Autodesk Inventor part; units mm, degrees
(part 6 of 8)
  arc A393 (19.9886, 4.7302) -> (19.9233, 4.7694) centre (19.956, 4.7498) ccw
  arc A394 (19.3814, 3.8663) -> (19.4467, 3.8271) centre (19.414, 3.8467) ccw
  line L135 (19.9559, 4.7498) -> (19.9559, 3.1242)
  arc A395 (19.9178, 3.1242) -> (19.994, 3.1242) centre (19.9559, 3.1242) ccw
  arc A396 (19.994, 4.7498) -> (19.9178, 4.7498) centre (19.9559, 4.7498) ccw
  line L136 (20.7656, 3.5758) -> (20.7656, 4.2982)
  arc A397 (20.8037, 4.2982) -> (20.7275, 4.2982) centre (20.7656, 4.2982) ccw
  arc A398 (20.7275, 3.5758) -> (20.8037, 3.5758) centre (20.7656, 3.5758) ccw
  arc A399 (21.6687, 4.2982) -> (20.7656, 4.2982) centre (21.2172, 4.2982) ccw
  arc A400 (21.6306, 4.2982) -> (21.7068, 4.2982) centre (21.6687, 4.2982) ccw
  arc A401 (20.7275, 4.2982) -> (20.8037, 4.2982) centre (20.7656, 4.2982) ccw
  line L137 (21.6687, 4.2982) -> (21.6687, 3.5758)
  arc A402 (21.6306, 3.5758) -> (21.7068, 3.5758) centre (21.6687, 3.5758) ccw
  arc A403 (21.7068, 4.2982) -> (21.6306, 4.2982) centre (21.6687, 4.2982) ccw
  arc A404 (20.7656, 3.5758) -> (21.6687, 3.5758) centre (21.2172, 3.5758) ccw
  arc A405 (20.8037, 3.5758) -> (20.7275, 3.5758) centre (20.7656, 3.5758) ccw
  arc A406 (21.7068, 3.5758) -> (21.6306, 3.5758) centre (21.6687, 3.5758) ccw
  line L138 (21.4881, 3.4854) -> (21.8493, 3.1242)
  arc A407 (21.8224, 3.0973) -> (21.8762, 3.1511) centre (21.8493, 3.1242) ccw
  arc A408 (21.515, 3.5124) -> (21.4611, 3.4585) centre (21.4881, 3.4855) ccw
  line L139 (22.6584, 4.7498) -> (22.2972, 3.4854)
  arc A409 (22.2605, 3.4959) -> (22.3338, 3.475) centre (22.2972, 3.4855) ccw
  arc A410 (22.6951, 4.7393) -> (22.6218, 4.7603) centre (22.6585, 4.7498) ccw
  line L140 (22.2972, 3.4854) -> (23.2003, 3.4854)
  arc A411 (23.2003, 3.4473) -> (23.2003, 3.5235) centre (23.2003, 3.4854) ccw
  arc A412 (22.2972, 3.5235) -> (22.2972, 3.4473) centre (22.2972, 3.4854) ccw
  line L141 (22.9293, 3.8467) -> (22.9293, 3.1242)
  arc A413 (22.8912, 3.1242) -> (22.9674, 3.1242) centre (22.9293, 3.1242) ccw
  arc A414 (22.9674, 3.8467) -> (22.8912, 3.8467) centre (22.9293, 3.8467) ccw
  line L142 (40.4622, 2.9972) -> (40.4622, 4.6228)
  arc A415 (40.5003, 4.6228) -> (40.4241, 4.6228) centre (40.4622, 4.6228) ccw
  arc A416 (40.4241, 2.9972) -> (40.5003, 2.9972) centre (40.4622, 2.9972) ccw
  line L143 (40.4622, 3.9003) -> (41.3653, 3.9003)
  arc A417 (41.3653, 3.8622) -> (41.3653, 3.9384) centre (41.3653, 3.9003) ccw
  arc A418 (40.4622, 3.9384) -> (40.4622, 3.8622) centre (40.4622, 3.9003) ccw
  line L144 (41.3653, 4.6228) -> (41.3653, 2.9972)
  arc A419 (41.3272, 2.9972) -> (41.4034, 2.9972) centre (41.3653, 2.9972) ccw
  arc A420 (41.4034, 4.6228) -> (41.3272, 4.6228) centre (41.3653, 4.6228) ccw
  line L145 (42.1295, 4.6228) -> (42.1295, 3.4488)
  arc A421 (42.0914, 3.4488) -> (42.1676, 3.4488) centre (42.1295, 3.4488) ccw
  arc A422 (42.1676, 4.6228) -> (42.0914, 4.6228) centre (42.1295, 4.6228) ccw
  arc A423 (42.1295, 3.4488) -> (43.0326, 3.4488) centre (42.5811, 3.4488) ccw
  arc A424 (42.1676, 3.4488) -> (42.0914, 3.4488) centre (42.1295, 3.4488) ccw
  arc A425 (43.0707, 3.4488) -> (42.9945, 3.4488) centre (43.0326, 3.4488) ccw
  line L146 (43.0326, 3.4488) -> (43.0326, 4.6228)
  arc A426 (43.0707, 4.6228) -> (42.9945, 4.6228) centre (43.0326, 4.6228) ccw
  arc A427 (42.9945, 3.4488) -> (43.0707, 3.4488) centre (43.0326, 3.4488) ccw
  line L147 (43.8108, 2.9972) -> (43.8108, 4.6228)
  arc A428 (43.8489, 4.6228) -> (43.7727, 4.6228) centre (43.8108, 4.6228) ccw
  arc A429 (43.7727, 2.9972) -> (43.8489, 2.9972) centre (43.8108, 2.9972) ccw
  line L148 (43.8108, 4.6228) -> (44.3526, 3.7197)
  arc A430 (44.32, 3.7001) -> (44.3853, 3.7393) centre (44.3527, 3.7197) ccw
  arc A431 (43.8434, 4.6424) -> (43.7781, 4.6032) centre (43.8107, 4.6228) ccw
  line L149 (44.3526, 3.7197) -> (44.8945, 4.6228)
  arc A432 (44.9272, 4.6032) -> (44.8618, 4.6424) centre (44.8945, 4.6228) ccw
  arc A433 (44.32, 3.7393) -> (44.3853, 3.7001) centre (44.3527, 3.7197) ccw
  line L150 (44.8945, 4.6228) -> (44.8945, 2.9972)
  arc A434 (44.8564, 2.9972) -> (44.9326, 2.9972) centre (44.8945, 2.9972) ccw
  arc A435 (44.9326, 4.6228) -> (44.8564, 4.6228) centre (44.8945, 4.6228) ccw
  line L151 (62.3062, 4.2418) -> (62.8481, 2.6162)
  arc A436 (62.8119, 2.6042) -> (62.8842, 2.6282) centre (62.8481, 2.6162) ccw
  arc A437 (62.3423, 4.2538) -> (62.2701, 4.2298) centre (62.3062, 4.2418) ccw
  line L152 (62.8481, 2.6162) -> (63.3899, 4.2418)
  arc A438 (63.4261, 4.2298) -> (63.3538, 4.2538) centre (63.3899, 4.2418) ccw
  arc A439 (62.8119, 2.6282) -> (62.8842, 2.6042) centre (62.8481, 2.6162) ccw
  line L153 (64.0986, 4.2418) -> (64.0986, 2.6162)
  arc A440 (64.0605, 2.6162) -> (64.1367, 2.6162) centre (64.0986, 2.6162) ccw
  arc A441 (64.1367, 4.2418) -> (64.0605, 4.2418) centre (64.0986, 4.2418) ccw
  line L154 (63.9179, 2.6162) -> (64.2792, 2.6162)
  arc A442 (64.2792, 2.5781) -> (64.2792, 2.6543) centre (64.2792, 2.6162) ccw
  arc A443 (63.9179, 2.6543) -> (63.9179, 2.5781) centre (63.9179, 2.6162) ccw
  line L155 (63.9179, 4.2418) -> (64.2792, 4.2418)
  arc A444 (64.2792, 4.2037) -> (64.2792, 4.2799) centre (64.2792, 4.2418) ccw
  arc A445 (63.9179, 4.2799) -> (63.9179, 4.2037) centre (63.9179, 4.2418) ccw
  line L156 (64.9707, 3.5193) -> (65.4223, 3.5193)
  arc A446 (65.4223, 3.4812) -> (65.4223, 3.5574) centre (65.4223, 3.5193) ccw
  arc A447 (64.9707, 3.5574) -> (64.9707, 3.4812) centre (64.9707, 3.5193) ccw
  arc A448 (65.4223, 2.6162) -> (65.4223, 3.5193) centre (65.4223, 3.0678) ccw
  arc A449 (65.4223, 2.6543) -> (65.4223, 2.5781) centre (65.4223, 2.6162) ccw
  arc A450 (65.4223, 3.5574) -> (65.4223, 3.4812) centre (65.4223, 3.5193) ccw
  line L157 (65.4223, 2.6162) -> (64.9707, 2.6162)
  arc A451 (64.9707, 2.6543) -> (64.9707, 2.5781) centre (64.9707, 2.6162) ccw
  arc A452 (65.4223, 2.5781) -> (65.4223, 2.6543) centre (65.4223, 2.6162) ccw
  line L158 (64.9707, 2.6162) -> (64.9707, 4.2418)
  arc A453 (65.0088, 4.2418) -> (64.9326, 4.2418) centre (64.9707, 4.2418) ccw
  arc A454 (64.9326, 2.6162) -> (65.0088, 2.6162) centre (64.9707, 2.6162) ccw
  line L159 (64.9707, 4.2418) -> (65.4223, 4.2418)
  arc A455 (65.4223, 4.2037) -> (65.4223, 4.2799) centre (65.4223, 4.2418) ccw
  arc A456 (64.9707, 4.2799) -> (64.9707, 4.2037) centre (64.9707, 4.2418) ccw
  arc A457 (65.4223, 3.5193) -> (65.4223, 4.2418) centre (65.4223, 3.8805) ccw
  arc A458 (65.4223, 3.5574) -> (65.4223, 3.4812) centre (65.4223, 3.5193) ccw
  arc A459 (65.4223, 4.2799) -> (65.4223, 4.2037) centre (65.4223, 4.2418) ccw
  arc A460 (84.4381, 2.6162) -> (84.7993, 2.9774) centre (84.4381, 2.9774) ccw
  arc A461 (84.4381, 2.6543) -> (84.4381, 2.5781) centre (84.4381, 2.6162) ccw
  arc A462 (84.8374, 2.9774) -> (84.7612, 2.9774) centre (84.7993, 2.9774) ccw
  arc A463 (83.8962, 2.842) -> (84.4381, 2.6162) centre (84.4381, 3.3794) ccw
  arc A464 (83.9233, 2.8688) -> (83.8691, 2.8151) centre (83.8962, 2.8419) ccw
  arc A465 (84.4381, 2.5781) -> (84.4381, 2.6543) centre (84.4381, 2.6162) ccw
  arc A466 (84.3026, 4.2418) -> (83.9414, 3.8806) centre (84.3026, 3.8806) ccw
  arc A467 (84.3026, 4.2037) -> (84.3026, 4.2799) centre (84.3026, 4.2418) ccw
  arc A468 (83.9033, 3.8806) -> (83.9795, 3.8806) centre (83.9414, 3.8806) ccw
  arc A469 (84.709, 4.1063) -> (84.3026, 4.2418) centre (84.3026, 3.5645) ccw
  arc A470 (84.6861, 4.0759) -> (84.7319, 4.1368) centre (84.709, 4.1063) ccw
  arc A471 (84.3026, 4.2799) -> (84.3026, 4.2037) centre (84.3026, 4.2418) ccw
  arc A472 (83.9414, 3.8806) -> (84.122, 3.5645) centre (84.3082, 3.8806) ccw
  arc A473 (83.9795, 3.8806) -> (83.9033, 3.8806) centre (83.9414, 3.8806) ccw
  arc A474 (84.1026, 3.5316) -> (84.1413, 3.5973) centre (84.1219, 3.5644) ccw
  arc A475 (84.7993, 2.9774) -> (84.6187, 3.2935) centre (84.4325, 2.9774) ccw
  arc A476 (84.7612, 2.9774) -> (84.8374, 2.9774) centre (84.7993, 2.9774) ccw
  arc A477 (84.638, 3.3264) -> (84.5993, 3.2607) centre (84.6187, 3.2936) ccw
  line L160 (84.6187, 3.2935) -> (84.122, 3.5645)
  arc A478 (84.1402, 3.5979) -> (84.1037, 3.531) centre (84.1219, 3.5644) ccw
  arc A479 (84.6004, 3.2601) -> (84.6369, 3.327) centre (84.6187, 3.2936) ccw
  line L161 (85.4623, 4.2418) -> (85.4623, 2.6162)
  arc A480 (85.4242, 2.6162) -> (85.5004, 2.6162) centre (85.4623, 2.6162) ccw
  arc A481 (85.5004, 4.2418) -> (85.4242, 4.2418) centre (85.4623, 4.2418) ccw
  line L162 (85.4623, 2.6162) -> (86.1848, 2.6162)
  arc A482 (86.1848, 2.5781) -> (86.1848, 2.6543) centre (86.1848, 2.6162) ccw
  arc A483 (85.4623, 2.6543) -> (85.4623, 2.5781) centre (85.4623, 2.6162) ccw
  line L163 (86.6716, 4.2418) -> (87.2135, 3.4742)
  arc A484 (87.1824, 3.4522) -> (87.2446, 3.4961) centre (87.2135, 3.4742) ccw
  arc A485 (86.7027, 4.2638) -> (86.6405, 4.2198) centre (86.6716, 4.2418) ccw
  line L164 (87.2135, 3.4742) -> (87.7553, 4.2418)
  arc A486 (87.7865, 4.2198) -> (87.7242, 4.2638) centre (87.7553, 4.2418) ccw
  arc A487 (87.1824, 3.4961) -> (87.2446, 3.4522) centre (87.2135, 3.4742) ccw
  line L165 (87.2135, 2.6162) -> (87.2135, 3.4742)
  arc A488 (87.2516, 3.4742) -> (87.1754, 3.4742) centre (87.2135, 3.4742) ccw
  arc A489 (87.1754, 2.6162) -> (87.2516, 2.6162) centre (87.2135, 2.6162) ccw
  line L166 (59.2187, 22.9362) -> (58.8574, 22.9362)
  arc A490 (58.8574, 22.9743) -> (58.8574, 22.8981) centre (58.8574, 22.9362) ccw
  arc A491 (59.2187, 22.8981) -> (59.2187, 22.9743) centre (59.2187, 22.9362) ccw
  arc A492 (58.4962, 23.2974) -> (58.8574, 22.9362) centre (58.8574, 23.2974) ccw
  arc A493 (58.5343, 23.2974) -> (58.4581, 23.2974) centre (58.4962, 23.2974) ccw
  arc A494 (58.8574, 22.8981) -> (58.8574, 22.9743) centre (58.8574, 22.9362) ccw
  line L167 (58.4962, 23.2974) -> (58.4962, 24.2006)
  arc A495 (58.5343, 24.2006) -> (58.4581, 24.2006) centre (58.4962, 24.2006) ccw
  arc A496 (58.4581, 23.2974) -> (58.5343, 23.2974) centre (58.4962, 23.2974) ccw
  arc A497 (58.8574, 24.5618) -> (58.4962, 24.2006) centre (58.8574, 24.2006) ccw
  arc A498 (58.8574, 24.5237) -> (58.8574, 24.5999) centre (58.8574, 24.5618) ccw
  arc A499 (58.4581, 24.2006) -> (58.5343, 24.2006) centre (58.4962, 24.2006) ccw
  line L168 (58.8574, 24.5618) -> (59.2187, 24.5618)
  arc A500 (59.2187, 24.5237) -> (59.2187, 24.5999) centre (59.2187, 24.5618) ccw
  arc A501 (58.8574, 24.5999) -> (58.8574, 24.5237) centre (58.8574, 24.5618) ccw
  line L169 (59.8028, 23.3878) -> (59.8028, 24.1102)
  arc A502 (59.8409, 24.1102) -> (59.7647, 24.1102) centre (59.8028, 24.1102) ccw
  arc A503 (59.7647, 23.3878) -> (59.8409, 23.3878) centre (59.8028, 23.3878) ccw
  arc A504 (60.7059, 24.1102) -> (59.8028, 24.1102) centre (60.2544, 24.1102) ccw
  arc A505 (60.6678, 24.1102) -> (60.744, 24.1102) centre (60.7059, 24.1102) ccw
  arc A506 (59.7647, 24.1102) -> (59.8409, 24.1102) centre (59.8028, 24.1102) ccw
  line L170 (60.7059, 24.1102) -> (60.7059, 23.3878)
  arc A507 (60.6678, 23.3878) -> (60.744, 23.3878) centre (60.7059, 23.3878) ccw
  arc A508 (60.744, 24.1102) -> (60.6678, 24.1102) centre (60.7059, 24.1102) ccw
  arc A509 (59.8027, 23.3878) -> (60.7059, 23.3878) centre (60.2543, 23.3878) ccw
  arc A510 (59.8408, 23.3878) -> (59.7646, 23.3878) centre (59.8027, 23.3878) ccw
  arc A511 (60.744, 23.3878) -> (60.6678, 23.3878) centre (60.7059, 23.3878) ccw
  line L171 (61.418, 22.9362) -> (61.418, 24.5618)
  arc A512 (61.4561, 24.5618) -> (61.3799, 24.5618) centre (61.418, 24.5618) ccw
  arc A513 (61.3799, 22.9362) -> (61.4561, 22.9362) centre (61.418, 22.9362) ccw
  line L172 (61.418, 24.5618) -> (62.3211, 22.9362)
  arc A514 (62.2878, 22.9177) -> (62.3544, 22.9547) centre (62.3211, 22.9362) ccw
  arc A515 (61.4513, 24.5803) -> (61.3847, 24.5433) centre (61.418, 24.5618) ccw
  line L173 (62.3211, 22.9362) -> (62.3211, 24.5618)
  arc A516 (62.3592, 24.5618) -> (62.283, 24.5618) centre (62.3211, 24.5618) ccw
  arc A517 (62.283, 22.9362) -> (62.3592, 22.9362) centre (62.3211, 22.9362) ccw
  line L174 (63.0853, 22.9362) -> (63.0853, 24.5618)
  arc A518 (63.1234, 24.5618) -> (63.0472, 24.5618) centre (63.0853, 24.5618) ccw
  arc A519 (63.0472, 22.9362) -> (63.1234, 22.9362) centre (63.0853, 22.9362) ccw
  line L175 (63.0853, 24.5618) -> (63.9884, 22.9362)
  arc A520 (63.9551, 22.9177) -> (64.0217, 22.9547) centre (63.9884, 22.9362) ccw
  arc A521 (63.1186, 24.5803) -> (63.052, 24.5433) centre (63.0853, 24.5618) ccw
  line L176 (63.9884, 22.9362) -> (63.9884, 24.5618)
  arc A522 (64.0265, 24.5618) -> (63.9503, 24.5618) centre (63.9884, 24.5618) ccw
  arc A523 (63.9503, 22.9362) -> (64.0265, 22.9362) centre (63.9884, 22.9362) ccw
  line L177 (65.4781, 22.9362) -> (64.7556, 22.9362)
  arc A524 (64.7556, 22.9743) -> (64.7556, 22.8981) centre (64.7556, 22.9362) ccw
  arc A525 (65.4781, 22.8981) -> (65.4781, 22.9743) centre (65.4781, 22.9362) ccw
  line L178 (64.7556, 22.9362) -> (64.7556, 24.5618)
  arc A526 (64.7937, 24.5618) -> (64.7175, 24.5618) centre (64.7556, 24.5618) ccw
  arc A527 (64.7175, 22.9362) -> (64.7937, 22.9362) centre (64.7556, 22.9362) ccw
  line L179 (64.7556, 24.5618) -> (65.4781, 24.5618)
  arc A528 (65.4781, 24.5237) -> (65.4781, 24.5999) centre (65.4781, 24.5618) ccw
  arc A529 (64.7556, 24.5999) -> (64.7556, 24.5237) centre (64.7556, 24.5618) ccw
  line L180 (64.7556, 23.8393) -> (65.2975, 23.8393)
  arc A530 (65.2975, 23.8012) -> (65.2975, 23.8774) centre (65.2975, 23.8393) ccw
  arc A531 (64.7556, 23.8774) -> (64.7556, 23.8012) centre (64.7556, 23.8393) ccw
  line L181 (66.7738, 22.9362) -> (66.4125, 22.9362)
  arc A532 (66.4125, 22.9743) -> (66.4125, 22.8981) centre (66.4125, 22.9362) ccw
  arc A533 (66.7738, 22.8981) -> (66.7738, 22.9743) centre (66.7738, 22.9362) ccw
  arc A534 (66.0513, 23.2974) -> (66.4125, 22.9362) centre (66.4125, 23.2974) ccw
  arc A535 (66.0894, 23.2974) -> (66.0132, 23.2974) centre (66.0513, 23.2974) ccw
  arc A536 (66.4125, 22.8981) -> (66.4125, 22.9743) centre (66.4125, 22.9362) ccw
  line L182 (66.0513, 23.2974) -> (66.0513, 24.2006)
  arc A537 (66.0894, 24.2006) -> (66.0132, 24.2006) centre (66.0513, 24.2006) ccw
  arc A538 (66.0132, 23.2974) -> (66.0894, 23.2974) centre (66.0513, 23.2974) ccw
  arc A539 (66.4125, 24.5618) -> (66.0513, 24.2006) centre (66.4125, 24.2006) ccw
  arc A540 (66.4125, 24.5237) -> (66.4125, 24.5999) centre (66.4125, 24.5618) ccw
  arc A541 (66.0132, 24.2006) -> (66.0894, 24.2006) centre (66.0513, 24.2006) ccw
  line L183 (66.4125, 24.5618) -> (66.7738, 24.5618)
  arc A542 (66.7738, 24.5237) -> (66.7738, 24.5999) centre (66.7738, 24.5618) ccw
  arc A543 (66.4125, 24.5999) -> (66.4125, 24.5237) centre (66.4125, 24.5618) ccw
  line L184 (67.7052, 22.9362) -> (67.7052, 24.5618)
  arc A544 (67.7433, 24.5618) -> (67.6671, 24.5618) centre (67.7052, 24.5618) ccw
  arc A545 (67.6671, 22.9362) -> (67.7433, 22.9362) centre (67.7052, 22.9362) ccw
  line L185 (67.2536, 24.5618) -> (68.1568, 24.5618)
  arc A546 (68.1568, 24.5237) -> (68.1568, 24.5999) centre (68.1568, 24.5618) ccw
  arc A547 (67.2536, 24.5999) -> (67.2536, 24.5237) centre (67.2536, 24.5618) ccw
  line L186 (68.7126, 23.3878) -> (68.7126, 24.1102)
  arc A548 (68.7507, 24.1102) -> (68.6745, 24.1102) centre (68.7126, 24.1102) ccw
  arc A549 (68.6745, 23.3878) -> (68.7507, 23.3878) centre (68.7126, 23.3878) ccw
  arc A550 (69.6157, 24.1102) -> (68.7126, 24.1102) centre (69.1642, 24.1102) ccw
  arc A551 (69.5776, 24.1102) -> (69.6538, 24.1102) centre (69.6157, 24.1102) ccw
  arc A552 (68.6745, 24.1102) -> (68.7507, 24.1102) centre (68.7126, 24.1102) ccw
  line L187 (69.6157, 24.1102) -> (69.6157, 23.3878)
  arc A553 (69.5776, 23.3878) -> (69.6538, 23.3878) centre (69.6157, 23.3878) ccw
  arc A554 (69.6538, 24.1102) -> (69.5776, 24.1102) centre (69.6157, 24.1102) ccw
  arc A555 (68.7126, 23.3878) -> (69.6157, 23.3878) centre (69.1642, 23.3878) ccw
  arc A556 (68.7507, 23.3878) -> (68.6745, 23.3878) centre (68.7126, 23.3878) ccw
  arc A557 (69.6538, 23.3878) -> (69.5776, 23.3878) centre (69.6157, 23.3878) ccw
  line L188 (70.3369, 22.9362) -> (70.3369, 24.5618)
  arc A558 (70.375, 24.5618) -> (70.2988, 24.5618) centre (70.3369, 24.5618) ccw
  arc A559 (70.2988, 22.9362) -> (70.375, 22.9362) centre (70.3369, 22.9362) ccw
  line L189 (70.3369, 24.5618) -> (70.7885, 24.5618)
  arc A560 (70.7885, 24.5237) -> (70.7885, 24.5999) centre (70.7885, 24.5618) ccw
  arc A561 (70.3369, 24.5999) -> (70.3369, 24.5237) centre (70.3369, 24.5618) ccw
  arc A562 (70.7885, 23.6587) -> (70.7885, 24.5618) centre (70.7885, 24.1103) ccw
  arc A563 (70.7885, 23.6968) -> (70.7885, 23.6206) centre (70.7885, 23.6587) ccw
  arc A564 (70.7885, 24.5999) -> (70.7885, 24.5237) centre (70.7885, 24.5618) ccw
  line L190 (70.7885, 23.6587) -> (70.3369, 23.6587)
  arc A565 (70.3369, 23.6968) -> (70.3369, 23.6206) centre (70.3369, 23.6587) ccw
  arc A566 (70.7885, 23.6206) -> (70.7885, 23.6968) centre (70.7885, 23.6587) ccw
  line L191 (71.24, 22.9362) -> (70.8788, 23.6587)
  arc A567 (70.9129, 23.6757) -> (70.8447, 23.6416) centre (70.8788, 23.6587) ccw
  arc A568 (71.206, 22.9192) -> (71.2741, 22.9532) centre (71.24, 22.9362) ccw
  arc A569 (72.3807, 22.9362) -> (72.7419, 23.2974) centre (72.3807, 23.2974) ccw
  arc A570 (72.3807, 22.9743) -> (72.3807, 22.8981) centre (72.3807, 22.9362) ccw
  arc A571 (72.78, 23.2974) -> (72.7038, 23.2974) centre (72.7419, 23.2974) ccw
  arc A572 (71.8388, 23.162) -> (72.3807, 22.9362) centre (72.3807, 23.6994) ccw
  arc A573 (71.8659, 23.1888) -> (71.8118, 23.1351) centre (71.8388, 23.1619) ccw
  arc A574 (72.3807, 22.8981) -> (72.3807, 22.9743) centre (72.3807, 22.9362) ccw
  arc A575 (72.2452, 24.5618) -> (71.884, 24.2006) centre (72.2452, 24.2006) ccw
  arc A576 (72.2452, 24.5237) -> (72.2452, 24.5999) centre (72.2452, 24.5618) ccw
  arc A577 (71.8459, 24.2006) -> (71.9221, 24.2006) centre (71.884, 24.2006) ccw
  arc A578 (72.6516, 24.4263) -> (72.2452, 24.5618) centre (72.2452, 23.8845) ccw
  arc A579 (72.6287, 24.3959) -> (72.6745, 24.4568) centre (72.6516, 24.4263) ccw
  arc A580 (72.2452, 24.5999) -> (72.2452, 24.5237) centre (72.2452, 24.5618) ccw
  arc A581 (71.884, 24.2006) -> (72.0646, 23.8845) centre (72.2508, 24.2006) ccw
  arc A582 (71.9221, 24.2006) -> (71.8459, 24.2006) centre (71.884, 24.2006) ccw
  arc A583 (72.0452, 23.8516) -> (72.0839, 23.9173) centre (72.0645, 23.8845) ccw
  arc A584 (72.7419, 23.2974) -> (72.5613, 23.6135) centre (72.3751, 23.2974) ccw
  arc A585 (72.7038, 23.2974) -> (72.78, 23.2974) centre (72.7419, 23.2974) ccw
  arc A586 (72.5806, 23.6464) -> (72.5419, 23.5807) centre (72.5613, 23.6136) ccw
  line L192 (72.5613, 23.6135) -> (72.0646, 23.8845)
  arc A587 (72.0828, 23.9179) -> (72.0463, 23.851) centre (72.0645, 23.8845) ccw
  arc A588 (72.543, 23.5801) -> (72.5795, 23.647) centre (72.5613, 23.6136) ccw
  line L193 (73.3498, 24.2006) -> (73.8014, 24.5618)
  arc A589 (73.8252, 24.532) -> (73.7776, 24.5916) centre (73.8014, 24.5618) ccw
  arc A590 (73.326, 24.2303) -> (73.3736, 24.1708) centre (73.3498, 24.2005) ccw
  line L194 (73.8014, 24.5618) -> (73.8014, 22.9362)
  arc A591 (73.7633, 22.9362) -> (73.8395, 22.9362) centre (73.8014, 22.9362) ccw
  arc A592 (73.8395, 24.5618) -> (73.7633, 24.5618) centre (73.8014, 24.5618) ccw
  line L195 (73.3498, 22.9362) -> (74.2529, 22.9362)
  arc A593 (74.2529, 22.8981) -> (74.2529, 22.9743) centre (74.2529, 22.9362) ccw
  arc A594 (73.3498, 22.9743) -> (73.3498, 22.8981) centre (73.3498, 22.9362) ccw
  line L196 (74.8469, 22.7556) -> (75.5694, 22.7556)
  arc A595 (75.5694, 22.7175) -> (75.5694, 22.7937) centre (75.5694, 22.7556) ccw
  arc A596 (74.8469, 22.7937) -> (74.8469, 22.7175) centre (74.8469, 22.7556) ccw
  arc A597 (76.6532, 22.9362) -> (77.0144, 23.2974) centre (76.6532, 23.2974) ccw
  arc A598 (76.6532, 22.9743) -> (76.6532, 22.8981) centre (76.6532, 22.9362) ccw
  arc A599 (77.0525, 23.2974) -> (76.9763, 23.2974) centre (77.0144, 23.2974) ccw
  arc A600 (76.1113, 23.162) -> (76.6532, 22.9362) centre (76.6532, 23.6994) ccw
  arc A601 (76.1384, 23.1888) -> (76.0843, 23.1351) centre (76.1113, 23.1619) ccw
  arc A602 (76.6532, 22.8981) -> (76.6532, 22.9743) centre (76.6532, 22.9362) ccw
  arc A603 (76.5177, 24.5618) -> (76.1565, 24.2006) centre (76.5177, 24.2006) ccw
  arc A604 (76.5177, 24.5237) -> (76.5177, 24.5999) centre (76.5177, 24.5618) ccw
  arc A605 (76.1184, 24.2006) -> (76.1946, 24.2006) centre (76.1565, 24.2006) ccw
  arc A606 (76.9241, 24.4263) -> (76.5177, 24.5618) centre (76.5177, 23.8845) ccw
  arc A607 (76.9013, 24.3959) -> (76.947, 24.4568) centre (76.9241, 24.4263) ccw
  arc A608 (76.5177, 24.5999) -> (76.5177, 24.5237) centre (76.5177, 24.5618) ccw
  arc A609 (76.1565, 24.2006) -> (76.3371, 23.8845) centre (76.5233, 24.2006) ccw
  arc A610 (76.1946, 24.2006) -> (76.1184, 24.2006) centre (76.1565, 24.2006) ccw
  arc A611 (76.3178, 23.8516) -> (76.3565, 23.9173) centre (76.3372, 23.8845) ccw
  arc A612 (77.0144, 23.2974) -> (76.8338, 23.6135) centre (76.6476, 23.2974) ccw
  arc A613 (76.9763, 23.2974) -> (77.0525, 23.2974) centre (77.0144, 23.2974) ccw
  arc A614 (76.8532, 23.6464) -> (76.8145, 23.5807) centre (76.8338, 23.6136) ccw
  line L197 (76.8338, 23.6135) -> (76.3371, 23.8845)
  arc A615 (76.3554, 23.9179) -> (76.3189, 23.851) centre (76.3372, 23.8845) ccw
  arc A616 (76.8156, 23.5801) -> (76.8521, 23.647) centre (76.8338, 23.6136) ccw
  line L198 (78.3999, 22.9362) -> (77.6774, 22.9362)
  arc A617 (77.6774, 22.9743) -> (77.6774, 22.8981) centre (77.6774, 22.9362) ccw
  arc A618 (78.3999, 22.8981) -> (78.3999, 22.9743) centre (78.3999, 22.9362) ccw
  line L199 (77.6774, 22.9362) -> (77.6774, 24.5618)
  arc A619 (77.7155, 24.5618) -> (77.6393, 24.5618) centre (77.6774, 24.5618) ccw
  arc A620 (77.6393, 22.9362) -> (77.7155, 22.9362) centre (77.6774, 22.9362) ccw
  line L200 (77.6774, 24.5618) -> (78.3999, 24.5618)
  arc A621 (78.3999, 24.5237) -> (78.3999, 24.5999) centre (78.3999, 24.5618) ccw
  arc A622 (77.6774, 24.5999) -> (77.6774, 24.5237) centre (77.6774, 24.5618) ccw
  line L201 (77.6774, 23.8393) -> (78.2193, 23.8393)
  arc A623 (78.2193, 23.8012) -> (78.2193, 23.8774) centre (78.2193, 23.8393) ccw
  arc A624 (77.6774, 23.8774) -> (77.6774, 23.8012) centre (77.6774, 23.8393) ccw
  line L202 (79.0292, 22.9362) -> (79.0292, 24.5618)
  arc A625 (79.0673, 24.5618) -> (78.9911, 24.5618) centre (79.0292, 24.5618) ccw
  arc A626 (78.9911, 22.9362) -> (79.0673, 22.9362) centre (79.0292, 22.9362) ccw
  line L203 (79.0292, 24.5618) -> (79.9323, 22.9362)
  arc A627 (79.899, 22.9177) -> (79.9656, 22.9547) centre (79.9323, 22.9362) ccw
  arc A628 (79.0625, 24.5803) -> (78.9959, 24.5433) centre (79.0292, 24.5618) ccw
  line L204 (79.9323, 22.9362) -> (79.9323, 24.5618)
  arc A629 (79.9704, 24.5618) -> (79.8942, 24.5618) centre (79.9323, 24.5618) ccw
  arc A630 (79.8942, 22.9362) -> (79.9704, 22.9362) centre (79.9323, 22.9362) ccw
  arc A631 (81.1342, 22.9362) -> (81.4954, 23.2974) centre (81.1342, 23.2974) ccw
  arc A632 (81.1342, 22.9743) -> (81.1342, 22.8981) centre (81.1342, 22.9362) ccw
  arc A633 (81.5335, 23.2974) -> (81.4573, 23.2974) centre (81.4954, 23.2974) ccw
  arc A634 (80.5923, 23.162) -> (81.1342, 22.9362) centre (81.1342, 23.6994) ccw
  arc A635 (80.6193, 23.1888) -> (80.5652, 23.1351) centre (80.5923, 23.162) ccw
  arc A636 (81.1342, 22.8981) -> (81.1342, 22.9743) centre (81.1342, 22.9362) ccw
  arc A637 (80.9987, 24.5618) -> (80.6374, 24.2006) centre (80.9987, 24.2005) ccw
  arc A638 (80.9987, 24.5237) -> (80.9987, 24.5999) centre (80.9987, 24.5618) ccw
  arc A639 (80.5993, 24.2006) -> (80.6755, 24.2006) centre (80.6374, 24.2006) ccw
  arc A640 (81.4051, 24.4263) -> (80.9987, 24.5618) centre (80.9987, 23.8845) ccw
  arc A641 (81.3822, 24.3959) -> (81.428, 24.4568) centre (81.4051, 24.4263) ccw
  arc A642 (80.9987, 24.5999) -> (80.9987, 24.5237) centre (80.9987, 24.5618) ccw
  arc A643 (80.6374, 24.2006) -> (80.8181, 23.8845) centre (81.0043, 24.2006) ccw
  arc A644 (80.6755, 24.2006) -> (80.5993, 24.2006) centre (80.6374, 24.2006) ccw
  arc A645 (80.7987, 23.8516) -> (80.8374, 23.9173) centre (80.8181, 23.8845) ccw
  arc A646 (81.4954, 23.2974) -> (81.3148, 23.6135) centre (81.1286, 23.2974) ccw
  arc A647 (81.4573, 23.2974) -> (81.5335, 23.2974) centre (81.4954, 23.2974) ccw
  arc A648 (81.3341, 23.6464) -> (81.2954, 23.5807) centre (81.3148, 23.6136) ccw
  line L205 (81.3148, 23.6135) -> (80.8181, 23.8845)
  arc A649 (80.8363, 23.9179) -> (80.7998, 23.851) centre (80.8181, 23.8845) ccw
  arc A650 (81.2965, 23.5801) -> (81.333, 23.647) centre (81.3148, 23.6136) ccw
  line L206 (82.1033, 23.3878) -> (82.1033, 24.1102)
  arc A651 (82.1414, 24.1102) -> (82.0652, 24.1102) centre (82.1033, 24.1102) ccw
  arc A652 (82.0652, 23.3878) -> (82.1414, 23.3878) centre (82.1033, 23.3878) ccw
  arc A653 (83.0064, 24.1102) -> (82.1033, 24.1102) centre (82.5549, 24.1102) ccw
  arc A654 (82.9683, 24.1102) -> (83.0445, 24.1102) centre (83.0064, 24.1102) ccw
  arc A655 (82.0652, 24.1102) -> (82.1414, 24.1102) centre (82.1033, 24.1102) ccw
  line L207 (83.0064, 24.1102) -> (83.0064, 23.3878)
  arc A656 (82.9683, 23.3878) -> (83.0445, 23.3878) centre (83.0064, 23.3878) ccw
  arc A657 (83.0445, 24.1102) -> (82.9683, 24.1102) centre (83.0064, 24.1102) ccw
  arc A658 (82.1033, 23.3878) -> (83.0064, 23.3878) centre (82.5549, 23.3878) ccw
  arc A659 (82.1414, 23.3878) -> (82.0652, 23.3878) centre (82.1033, 23.3878) ccw
  arc A660 (83.0445, 23.3878) -> (82.9683, 23.3878) centre (83.0064, 23.3878) ccw
  arc A661 (29.4833, 24.1102) -> (29.5595, 24.1102) centre (29.5214, 24.1102) ccw
  arc A662 (30.3864, 24.1102) -> (30.4626, 24.1102) centre (30.4245, 24.1102) ccw
  arc A663 (30.4245, 24.1102) -> (29.5214, 24.1102) centre (29.9729, 24.1102) ccw
  arc A664 (29.4833, 23.3878) -> (29.5595, 23.3878) centre (29.5214, 23.3878) ccw
  arc A665 (29.5595, 24.1102) -> (29.4833, 24.1102) centre (29.5214, 24.1102) ccw
  line L208 (29.5214, 23.3878) -> (29.5214, 24.1102)
  arc A666 (28.483, 24.5999) -> (28.483, 24.5237) centre (28.483, 24.5618) ccw
  arc A667 (28.483, 23.8774) -> (28.483, 23.8012) centre (28.483, 23.8393) ccw
  arc A668 (28.483, 23.8393) -> (28.483, 24.5618) centre (28.483, 24.2005) ccw
  arc A669 (28.0315, 24.5999) -> (28.0315, 24.5237) centre (28.0315, 24.5618) ccw
  arc A670 (28.483, 24.5237) -> (28.483, 24.5999) centre (28.483, 24.5618) ccw
  line L209 (28.0315, 24.5618) -> (28.483, 24.5618)
  arc A671 (27.9934, 22.9362) -> (28.0696, 22.9362) centre (28.0315, 22.9362) ccw
  arc A672 (28.0696, 24.5618) -> (27.9934, 24.5618) centre (28.0315, 24.5618) ccw
  line L210 (28.0315, 22.9362) -> (28.0315, 24.5618)
  arc A673 (28.483, 22.8981) -> (28.483, 22.9743) centre (28.483, 22.9362) ccw
  arc A674 (28.0315, 22.9743) -> (28.0315, 22.8981) centre (28.0315, 22.9362) ccw
  line L211 (28.483, 22.9362) -> (28.0315, 22.9362)
  arc A675 (28.483, 23.8774) -> (28.483, 23.8012) centre (28.483, 23.8393) ccw
  arc A676 (28.483, 22.9743) -> (28.483, 22.8981) centre (28.483, 22.9362) ccw
  arc A677 (28.483, 22.9362) -> (28.483, 23.8393) centre (28.483, 23.3878) ccw
  arc A678 (28.0315, 23.8774) -> (28.0315, 23.8012) centre (28.0315, 23.8393) ccw
  arc A679 (28.483, 23.8012) -> (28.483, 23.8774) centre (28.483, 23.8393) ccw
  line L212 (28.0315, 23.8393) -> (28.483, 23.8393)
  arc A680 (27.3364, 23.3878) -> (27.2602, 23.3878) centre (27.2983, 23.3878) ccw
  arc A681 (26.4333, 23.3878) -> (26.3571, 23.3878) centre (26.3952, 23.3878) ccw
  arc A682 (26.3952, 23.3878) -> (27.2983, 23.3878) centre (26.8468, 23.3878) ccw
  arc A683 (27.3364, 24.1102) -> (27.2602, 24.1102) centre (27.2983, 24.1102) ccw
  arc A684 (27.2602, 23.3878) -> (27.3364, 23.3878) centre (27.2983, 23.3878) ccw
  line L213 (27.2983, 24.1102) -> (27.2983, 23.3878)
  arc A685 (26.3571, 24.1102) -> (26.4333, 24.1102) centre (26.3952, 24.1102) ccw
  arc A686 (27.2602, 24.1102) -> (27.3364, 24.1102) centre (27.2983, 24.1102) ccw
  arc A687 (27.2983, 24.1102) -> (26.3952, 24.1102) centre (26.8468, 24.1102) ccw
  arc A688 (26.3571, 23.3878) -> (26.4333, 23.3878) centre (26.3952, 23.3878) ccw
  arc A689 (26.4333, 24.1102) -> (26.3571, 24.1102) centre (26.3952, 24.1102) ccw
  line L214 (26.3952, 23.3878) -> (26.3952, 24.1102)
  arc A690 (25.7102, 22.9192) -> (25.7784, 22.9532) centre (25.7443, 22.9362) ccw
  arc A691 (25.4171, 23.6757) -> (25.349, 23.6416) centre (25.3831, 23.6587) ccw
  line L215 (25.7443, 22.9362) -> (25.3831, 23.6587)
  arc A692 (25.2928, 23.6206) -> (25.2928, 23.6968) centre (25.2928, 23.6587) ccw
  arc A693 (24.8412, 23.6968) -> (24.8412, 23.6206) centre (24.8412, 23.6587) ccw
  line L216 (25.2928, 23.6587) -> (24.8412, 23.6587)
  arc A694 (25.2928, 24.5999) -> (25.2928, 24.5237) centre (25.2928, 24.5618) ccw
  arc A695 (25.2928, 23.6968) -> (25.2928, 23.6206) centre (25.2928, 23.6587) ccw
  arc A696 (25.2928, 23.6587) -> (25.2928, 24.5618) centre (25.2928, 24.1103) ccw
  arc A697 (24.8412, 24.5999) -> (24.8412, 24.5237) centre (24.8412, 24.5618) ccw
  arc A698 (25.2928, 24.5237) -> (25.2928, 24.5999) centre (25.2928, 24.5618) ccw
  line L217 (24.8412, 24.5618) -> (25.2928, 24.5618)
  arc A699 (24.8031, 22.9362) -> (24.8793, 22.9362) centre (24.8412, 22.9362) ccw
  arc A700 (24.8793, 24.5618) -> (24.8031, 24.5618) centre (24.8412, 24.5618) ccw
  line L218 (24.8412, 22.9362) -> (24.8412, 24.5618)
  arc A701 (88.3801, 23.3045) -> (88.3801, 23.3807) centre (88.3801, 23.3426) ccw
  arc A702 (87.5673, 23.3807) -> (87.5673, 23.3045) centre (87.5673, 23.3426) ccw
  line L219 (88.3801, 23.3426) -> (87.5673, 23.3426)
  arc A703 (88.0098, 24.5738) -> (87.9375, 24.5498) centre (87.9736, 24.5618) ccw
  arc A704 (88.4794, 22.9242) -> (88.5517, 22.9482) centre (88.5155, 22.9362) ccw
  line L220 (87.9737, 24.5618) -> (88.5156, 22.9362)
  arc A705 (87.3957, 22.9482) -> (87.468, 22.9242) centre (87.4318, 22.9362) ccw
  arc A706 (88.0098, 24.5498) -> (87.9375, 24.5738) centre (87.9736, 24.5618) ccw
  line L221 (87.4318, 22.9362) -> (87.9737, 24.5618)
  arc A707 (86.5768, 24.5999) -> (86.5768, 24.5237) centre (86.5768, 24.5618) ccw
  arc A708 (86.9381, 24.5237) -> (86.9381, 24.5999) centre (86.9381, 24.5618) ccw
  line L222 (86.5768, 24.5618) -> (86.9381, 24.5618)
  arc A709 (86.1775, 24.2006) -> (86.2537, 24.2006) centre (86.2156, 24.2006) ccw
  arc A710 (86.5768, 24.5237) -> (86.5768, 24.5999) centre (86.5768, 24.5618) ccw
  arc A711 (86.5768, 24.5618) -> (86.2156, 24.2006) centre (86.5768, 24.2006) ccw
  arc A712 (86.1775, 23.2974) -> (86.2537, 23.2974) centre (86.2156, 23.2974) ccw
  arc A713 (86.2537, 24.2006) -> (86.1775, 24.2006) centre (86.2156, 24.2006) ccw
  line L223 (86.2156, 23.2974) -> (86.2156, 24.2006)
  arc A714 (86.5768, 22.8981) -> (86.5768, 22.9743) centre (86.5768, 22.9362) ccw
  arc A715 (86.2537, 23.2974) -> (86.1775, 23.2974) centre (86.2156, 23.2974) ccw
  arc A716 (86.2156, 23.2974) -> (86.5768, 22.9362) centre (86.5768, 23.2974) ccw
  arc A717 (86.9381, 22.8981) -> (86.9381, 22.9743) centre (86.9381, 22.9362) ccw
  arc A718 (86.5768, 22.9743) -> (86.5768, 22.8981) centre (86.5768, 22.9362) ccw
  line L224 (86.9381, 22.9362) -> (86.5768, 22.9362)
  arc A719 (85.24, 24.5999) -> (85.24, 24.5237) centre (85.24, 24.5618) ccw
  arc A720 (85.6012, 24.5237) -> (85.6012, 24.5999) centre (85.6012, 24.5618) ccw
  line L225 (85.24, 24.5618) -> (85.6012, 24.5618)
  arc A721 (85.24, 22.9743) -> (85.24, 22.8981) centre (85.24, 22.9362) ccw
  arc A722 (85.6012, 22.8981) -> (85.6012, 22.9743) centre (85.6012, 22.9362) ccw
  line L226 (85.24, 22.9362) -> (85.6012, 22.9362)
  arc A723 (85.4587, 24.5618) -> (85.3825, 24.5618) centre (85.4206, 24.5618) ccw
  arc A724 (85.3825, 22.9362) -> (85.4587, 22.9362) centre (85.4206, 22.9362) ccw
  line L227 (85.4206, 24.5618) -> (85.4206, 22.9362)
  arc A725 (84.5967, 22.9192) -> (84.6649, 22.9532) centre (84.6308, 22.9362) ccw
  arc A726 (84.3036, 23.6757) -> (84.2355, 23.6416) centre (84.2696, 23.6587) ccw
  line L228 (84.6308, 22.9362) -> (84.2696, 23.6587)
  arc A727 (84.1792, 23.6206) -> (84.1792, 23.6968) centre (84.1792, 23.6587) ccw
  arc A728 (83.7277, 23.6968) -> (83.7277, 23.6206) centre (83.7277, 23.6587) ccw
  line L229 (84.1792, 23.6587) -> (83.7277, 23.6587)
  arc A729 (84.1792, 24.5999) -> (84.1792, 24.5237) centre (84.1792, 24.5618) ccw
  arc A730 (84.1792, 23.6968) -> (84.1792, 23.6206) centre (84.1792, 23.6587) ccw
  arc A731 (84.1792, 23.6587) -> (84.1792, 24.5618) centre (84.1792, 24.1103) ccw
  arc A732 (83.7277, 24.5999) -> (83.7277, 24.5237) centre (83.7277, 24.5618) ccw
  arc A733 (84.1792, 24.5237) -> (84.1792, 24.5999) centre (84.1792, 24.5618) ccw
  line L230 (83.7277, 24.5618) -> (84.1792, 24.5618)
  arc A734 (83.6896, 22.9362) -> (83.7658, 22.9362) centre (83.7277, 22.9362) ccw
  arc A735 (83.7658, 24.5618) -> (83.6896, 24.5618) centre (83.7277, 24.5618) ccw
  line L231 (83.7277, 22.9362) -> (83.7277, 24.5618)
  arc A736 (14.1986, 26.9875) -> (14.4526, 27.2415) centre (14.1986, 27.2415) ccw
  arc A737 (14.1986, 27.0192) -> (14.1986, 26.9558) centre (14.1986, 26.9875) ccw
  arc A738 (14.4844, 27.2415) -> (14.4208, 27.2415) centre (14.4526, 27.2415) ccw
  arc A739 (13.8176, 27.1463) -> (14.1986, 26.9875) centre (14.1987, 27.5241) ccw
  arc A740 (13.8401, 27.1686) -> (13.7951, 27.1239) centre (13.8176, 27.1463) ccw
  arc A741 (14.1986, 26.9558) -> (14.1986, 27.0192) centre (14.1986, 26.9875) ccw
  arc A742 (14.1034, 28.1305) -> (13.8494, 27.8765) centre (14.1034, 27.8765) ccw
  arc A743 (14.1034, 28.0988) -> (14.1034, 28.1623) centre (14.1034, 28.1306) ccw
  arc A744 (13.8176, 27.8765) -> (13.8811, 27.8765) centre (13.8494, 27.8765) ccw
  arc A745 (14.3891, 28.0353) -> (14.1034, 28.1305) centre (14.1035, 27.6544) ccw
  arc A746 (14.37, 28.0099) -> (14.4082, 28.0606) centre (14.3891, 28.0353) ccw
  arc A747 (14.1033, 28.1623) -> (14.1034, 28.0988) centre (14.1034, 28.1306) ccw
  arc A748 (13.8494, 27.8765) -> (13.9764, 27.6543) centre (14.1073, 27.8765) ccw
  arc A749 (13.8811, 27.8765) -> (13.8176, 27.8765) centre (13.8494, 27.8765) ccw
  arc A750 (13.9602, 27.6269) -> (13.9925, 27.6816) centre (13.9764, 27.6543) ccw
  arc A751 (14.4526, 27.2415) -> (14.3256, 27.4638) centre (14.1946, 27.2415) ccw
  arc A752 (14.4208, 27.2415) -> (14.4844, 27.2415) centre (14.4526, 27.2415) ccw
  arc A753 (14.3417, 27.4911) -> (14.3095, 27.4364) centre (14.3256, 27.4638) ccw
  line L232 (14.3256, 27.4638) -> (13.9764, 27.6543)
  arc A754 (13.9916, 27.6821) -> (13.9611, 27.6264) centre (13.9764, 27.6543) ccw
  arc A755 (14.3104, 27.4359) -> (14.3408, 27.4916) centre (14.3256, 27.4638) ccw
  line L233 (14.859, 28.1305) -> (15.24, 26.9875)
  arc A756 (15.2099, 26.9775) -> (15.2701, 26.9975) centre (15.24, 26.9875) ccw
  arc A757 (14.8891, 28.1405) -> (14.8289, 28.1205) centre (14.859, 28.1305) ccw
  line L234 (15.24, 26.9875) -> (15.621, 28.1305)
  arc A758 (15.6511, 28.1205) -> (15.5909, 28.1405) centre (15.621, 28.1305) ccw
  arc A759 (15.2099, 26.9975) -> (15.2701, 26.9775) centre (15.24, 26.9875) ccw
  line L235 (16.0655, 27.8765) -> (16.383, 28.1305)
  arc A760 (16.4028, 28.1057) -> (16.3632, 28.1553) centre (16.383, 28.1305) ccw
  arc A761 (32.5995, 30.1046) -> (32.5487, 30.1046) centre (32.5741, 30.1046) ccw
  arc A762 (16.0457, 27.9013) -> (16.0853, 27.8517) centre (16.0655, 27.8765) ccw
  line L236 (16.383, 28.1305) -> (16.383, 26.9875)
  arc A763 (16.3513, 26.9875) -> (16.4147, 26.9875) centre (16.383, 26.9875) ccw
  arc A764 (16.4147, 28.1305) -> (16.3513, 28.1305) centre (16.383, 28.1305) ccw
  line L237 (16.0655, 26.9875) -> (16.7005, 26.9875)
  arc A765 (16.7005, 26.9558) -> (16.7005, 27.0192) centre (16.7005, 26.9875) ccw
  arc A766 (16.0655, 27.0192) -> (16.0655, 26.9558) centre (16.0655, 26.9875) ccw
  arc A767 (58.219, 30.4546) -> (58.219, 30.4038) centre (58.219, 30.4292) ccw
  arc A768 (32.5487, 29.5854) -> (32.5995, 29.5854) centre (32.5741, 29.5854) ccw
  arc A769 (49.8475, 27.1145) -> (50.1015, 27.3685) centre (49.8475, 27.3685) ccw
  arc A770 (49.8475, 27.1462) -> (49.8475, 27.0828) centre (49.8475, 27.1145) ccw
  arc A771 (50.1333, 27.3685) -> (50.0697, 27.3685) centre (50.1015, 27.3685) ccw
  arc A772 (49.4665, 27.2733) -> (49.8475, 27.1145) centre (49.8476, 27.6511) ccw
  arc A773 (49.489, 27.2956) -> (49.444, 27.2509) centre (49.4665, 27.2733) ccw
  arc A774 (49.8475, 27.0828) -> (49.8475, 27.1462) centre (49.8475, 27.1145) ccw
  arc A775 (49.7523, 28.2575) -> (49.4983, 28.0035) centre (49.7523, 28.0035) ccw
  arc A776 (49.7523, 28.2258) -> (49.7523, 28.2892) centre (49.7523, 28.2575) ccw
  arc A777 (49.4665, 28.0035) -> (49.53, 28.0035) centre (49.4983, 28.0035) ccw
  arc A778 (50.038, 28.1623) -> (49.7523, 28.2575) centre (49.7524, 27.7814) ccw
  arc A779 (50.0189, 28.1369) -> (50.0571, 28.1876) centre (50.038, 28.1623) ccw
  arc A780 (49.7522, 28.2892) -> (49.7523, 28.2258) centre (49.7523, 28.2575) ccw
  arc A781 (49.4983, 28.0035) -> (49.6253, 27.7813) centre (49.7562, 28.0035) ccw
  arc A782 (49.53, 28.0035) -> (49.4665, 28.0035) centre (49.4983, 28.0035) ccw
  arc A783 (49.6091, 27.7539) -> (49.6414, 27.8086) centre (49.6252, 27.7812) ccw
  arc A784 (50.1015, 27.3685) -> (49.9745, 27.5907) centre (49.8436, 27.3685) ccw
  arc A785 (50.0697, 27.3685) -> (50.1333, 27.3685) centre (50.1015, 27.3685) ccw
  arc A786 (49.9906, 27.6181) -> (49.9584, 27.5634) centre (49.9745, 27.5907) ccw
  line L238 (49.9745, 27.5907) -> (49.6253, 27.7813)
  arc A787 (49.6405, 27.8091) -> (49.61, 27.7534) centre (49.6252, 27.7812) ccw
  arc A788 (49.9593, 27.5629) -> (49.9897, 27.6186) centre (49.9745, 27.5907) ccw
  line L239 (50.5079, 28.2575) -> (50.8889, 27.1145)
  arc A789 (50.8588, 27.1045) -> (50.919, 27.1245) centre (50.8889, 27.1145) ccw
  arc A790 (50.538, 28.2675) -> (50.4778, 28.2475) centre (50.5079, 28.2575) ccw
  line L240 (50.8889, 27.1145) -> (51.2699, 28.2575)
  arc A791 (51.3, 28.2475) -> (51.2398, 28.2675) centre (51.2699, 28.2575) ccw
  arc A792 (50.8588, 27.1245) -> (50.919, 27.1045) centre (50.8889, 27.1145) ccw
  arc A793 (52.3494, 27.9718) -> (52.0637, 28.2575) centre (52.0637, 27.9718) ccw
  arc A794 (52.3177, 27.9718) -> (52.3812, 27.9718) centre (52.3494, 27.9718) ccw
  arc A795 (52.0637, 28.2892) -> (52.0637, 28.2258) centre (52.0637, 28.2575) ccw
  arc A796 (52.0637, 28.2575) -> (51.7144, 28.0035) centre (52.0637, 27.8904) ccw
  arc A797 (52.0636, 28.2258) -> (52.0637, 28.2892) centre (52.0637, 28.2575) ccw
  arc A798 (51.6842, 28.0133) -> (51.7446, 27.9937) centre (51.7144, 28.0035) ccw
  arc A799 (52.2542, 27.7495) -> (52.3494, 27.9718) centre (52.0425, 27.9717) ccw
  arc A800 (52.2323, 27.7725) -> (52.276, 27.7265) centre (52.2542, 27.7495) ccw
  arc A801 (52.3811, 27.9718) -> (52.3177, 27.9717) centre (52.3494, 27.9718) ccw
  line L241 (52.2542, 27.7495) -> (51.7144, 27.1145)
  arc A802 (51.6902, 27.1351) -> (51.7386, 27.0939) centre (51.7144, 27.1145) ccw
  arc A803 (52.2783, 27.7289) -> (52.23, 27.7701) centre (52.2542, 27.7495) ccw
  line L242 (51.7144, 27.1145) -> (52.3494, 27.1145)
  arc A804 (52.3494, 27.0828) -> (52.3494, 27.1462) centre (52.3494, 27.1145) ccw
  arc A805 (51.7144, 27.1462) -> (51.7144, 27.0828) centre (51.7144, 27.1145) ccw
  arc A806 (32.5995, 29.5854) -> (32.5487, 29.5854) centre (32.5741, 29.5854) ccw
  arc A807 (33.2486, 29.5854) -> (33.1978, 29.5854) centre (33.2232, 29.5854) ccw
  line L243 (33.7552, 30.4292) -> (33.7552, 29.5854)
  arc A808 (33.7298, 29.5854) -> (33.7806, 29.5854) centre (33.7552, 29.5854) ccw
  arc A809 (33.7806, 30.4292) -> (33.7298, 30.4292) centre (33.7552, 30.4292) ccw
  arc A810 (33.7552, 29.5854) -> (34.4043, 29.5854) centre (34.0798, 29.5854) ccw
  arc A811 (33.7806, 29.5854) -> (33.7298, 29.5854) centre (33.7552, 29.5854) ccw
  arc A812 (34.4297, 29.5854) -> (34.3789, 29.5854) centre (34.4043, 29.5854) ccw
  line L244 (34.4043, 29.5854) -> (34.4043, 30.4292)
  arc A813 (34.4297, 30.4292) -> (34.3789, 30.4292) centre (34.4043, 30.4292) ccw
  arc A814 (34.3789, 29.5854) -> (34.4297, 29.5854) centre (34.4043, 29.5854) ccw
  line L245 (35.1846, 29.2608) -> (35.1846, 30.4292)
  arc A815 (35.21, 30.4292) -> (35.1592, 30.4292) centre (35.1846, 30.4292) ccw
  arc A816 (35.1592, 29.2608) -> (35.21, 29.2608) centre (35.1846, 29.2608) ccw
  line L246 (34.8601, 30.4292) -> (35.5092, 30.4292)
  arc A817 (35.5092, 30.4038) -> (35.5092, 30.4546) centre (35.5092, 30.4292) ccw
  arc A818 (34.8601, 30.4546) -> (34.8601, 30.4038) centre (34.8601, 30.4292) ccw
  arc A819 (33.2232, 30.1046) -> (32.5741, 30.1046) centre (32.8987, 30.1046) ccw
  arc A820 (33.1978, 30.1046) -> (33.2486, 30.1046) centre (33.2232, 30.1046) ccw
  arc A821 (32.5487, 30.1046) -> (32.5995, 30.1046) centre (32.5741, 30.1046) ccw
  line L247 (33.2232, 30.1046) -> (33.2232, 29.5854)
  arc A822 (33.1978, 29.5854) -> (33.2486, 29.5854) centre (33.2232, 29.5854) ccw
  arc A823 (33.2486, 30.1046) -> (33.1978, 30.1046) centre (33.2232, 30.1046) ccw
  arc A824 (32.5741, 29.5854) -> (33.2232, 29.5854) centre (32.8987, 29.5854) ccw
  line L248 (32.5741, 29.5854) -> (32.5741, 30.1046)
  arc A825 (32.0167, 29.2608) -> (32.0675, 29.2608) centre (32.0421, 29.2608) ccw
  arc A826 (32.0675, 30.4292) -> (32.0167, 30.4292) centre (32.0421, 30.4292) ccw
  line L249 (32.0421, 29.2608) -> (32.0421, 30.4292)
  arc A827 (31.4152, 30.4415) -> (31.3708, 30.4169) centre (31.393, 30.4292) ccw
  arc A828 (32.0199, 29.2485) -> (32.0643, 29.2731) centre (32.0421, 29.2608) ccw
  line L250 (31.393, 30.4292) -> (32.0421, 29.2608)
  arc A829 (31.3676, 29.2608) -> (31.4184, 29.2608) centre (31.393, 29.2608) ccw
  arc A830 (31.4184, 30.4292) -> (31.3676, 30.4292) centre (31.393, 30.4292) ccw
  line L251 (31.393, 29.2608) -> (31.393, 30.4292)
  arc A831 (30.6352, 30.4546) -> (30.6352, 30.4038) centre (30.6352, 30.4292) ccw
  arc A832 (30.8949, 30.4038) -> (30.8949, 30.4546) centre (30.8949, 30.4292) ccw
  line L252 (30.6352, 30.4292) -> (30.8949, 30.4292)
  arc A833 (30.6352, 29.2862) -> (30.6352, 29.2354) centre (30.6352, 29.2608) ccw
  arc A834 (30.8949, 29.2354) -> (30.8949, 29.2862) centre (30.8949, 29.2608) ccw
  line L253 (30.6352, 29.2608) -> (30.8949, 29.2608)
  arc A835 (30.7905, 30.4292) -> (30.7397, 30.4292) centre (30.7651, 30.4292) ccw
  arc A836 (30.7397, 29.2608) -> (30.7905, 29.2608) centre (30.7651, 29.2608) ccw
  line L254 (30.7651, 30.4292) -> (30.7651, 29.2608)
  arc A837 (30.1117, 29.5854) -> (30.1625, 29.5854) centre (30.1371, 29.5854) ccw
  arc A838 (30.1625, 30.4292) -> (30.1117, 30.4292) centre (30.1371, 30.4292) ccw
  line L255 (30.1371, 29.5854) -> (30.1371, 30.4292)
  arc A839 (30.1625, 29.5854) -> (30.1117, 29.5854) centre (30.1371, 29.5854) ccw
  arc A840 (29.5134, 29.5854) -> (29.4626, 29.5854) centre (29.488, 29.5854) ccw
  arc A841 (29.488, 29.5854) -> (30.1371, 29.5854) centre (29.8126, 29.5854) ccw
  arc A842 (29.5134, 30.4292) -> (29.4626, 30.4292) centre (29.488, 30.4292) ccw
  arc A843 (29.4626, 29.5854) -> (29.5134, 29.5854) centre (29.488, 29.5854) ccw
  line L256 (29.488, 30.4292) -> (29.488, 29.5854)
  arc A844 (28.5934, 29.2354) -> (28.5934, 29.2862) centre (28.5934, 29.2608) ccw
  arc A845 (28.2688, 29.2862) -> (28.2688, 29.2354) centre (28.2688, 29.2608) ccw
  line L257 (28.5934, 29.2608) -> (28.2688, 29.2608)
  arc A846 (28.9433, 29.5854) -> (28.8925, 29.5854) centre (28.9179, 29.5854) ccw
  arc A847 (28.5934, 29.2862) -> (28.5934, 29.2354) centre (28.5934, 29.2608) ccw
  arc A848 (28.5934, 29.2608) -> (28.9179, 29.5854) centre (28.5933, 29.5854) ccw
  arc A849 (28.9433, 30.1046) -> (28.8925, 30.1046) centre (28.9179, 30.1046) ccw
  arc A850 (28.8925, 29.5854) -> (28.9433, 29.5854) centre (28.9179, 29.5854) ccw
  line L258 (28.9179, 30.1046) -> (28.9179, 29.5854)
  arc A851 (28.5934, 30.4546) -> (28.5934, 30.4038) centre (28.5934, 30.4292) ccw
  arc A852 (28.8925, 30.1046) -> (28.9433, 30.1046) centre (28.9179, 30.1046) ccw
  arc A853 (28.9179, 30.1046) -> (28.5934, 30.4292) centre (28.5933, 30.1046) ccw
  arc A854 (28.2688, 30.4546) -> (28.2688, 30.4038) centre (28.2688, 30.4292) ccw
  arc A855 (28.5934, 30.4038) -> (28.5934, 30.4546) centre (28.5934, 30.4292) ccw
  line L259 (28.2688, 30.4292) -> (28.5934, 30.4292)
  arc A856 (28.2434, 29.2608) -> (28.2942, 29.2608) centre (28.2688, 29.2608) ccw
  arc A857 (28.2942, 30.4292) -> (28.2434, 30.4292) centre (28.2688, 30.4292) ccw
  line L260 (28.2688, 29.2608) -> (28.2688, 30.4292)
  arc A858 (27.7215, 29.2494) -> (27.7669, 29.2722) centre (27.7442, 29.2608) ccw
  arc A859 (27.5073, 29.7914) -> (27.4618, 29.7687) centre (27.4845, 29.78) ccw
  line L261 (27.7442, 29.2608) -> (27.4845, 29.7801)
  arc A860 (27.4196, 29.7547) -> (27.4196, 29.8055) centre (27.4196, 29.7801) ccw
  arc A861 (27.0951, 29.8055) -> (27.0951, 29.7547) centre (27.0951, 29.7801) ccw
  line L262 (27.4196, 29.7801) -> (27.0951, 29.7801)
  arc A862 (27.4196, 30.4546) -> (27.4196, 30.4038) centre (27.4196, 30.4292) ccw
  arc A863 (27.4196, 29.8055) -> (27.4196, 29.7547) centre (27.4196, 29.7801) ccw
  arc A864 (27.4196, 29.7801) -> (27.4196, 30.4292) centre (27.4196, 30.1046) ccw
  arc A865 (27.0951, 30.4546) -> (27.0951, 30.4038) centre (27.0951, 30.4292) ccw
  arc A866 (27.4196, 30.4038) -> (27.4196, 30.4546) centre (27.4196, 30.4292) ccw
  line L263 (27.0951, 30.4292) -> (27.4196, 30.4292)
  arc A867 (27.0697, 29.2608) -> (27.1205, 29.2608) centre (27.0951, 29.2608) ccw
  arc A868 (27.1205, 30.4292) -> (27.0697, 30.4292) centre (27.0951, 30.4292) ccw
  line L264 (27.0951, 29.2608) -> (27.0951, 30.4292)
  arc A869 (26.5233, 29.5275) -> (26.5233, 29.5783) centre (26.5233, 29.5529) ccw
  arc A870 (25.9391, 29.5783) -> (25.9391, 29.5275) centre (25.9391, 29.5529) ccw
  line L265 (26.5233, 29.5529) -> (25.9391, 29.5529)
  arc A871 (26.2553, 30.4372) -> (26.2071, 30.4212) centre (26.2312, 30.4292) ccw
  arc A872 (26.5965, 29.2528) -> (26.6447, 29.2688) centre (26.6206, 29.2608) ccw
  line L266 (26.2312, 30.4292) -> (26.6206, 29.2608)
  arc A873 (25.8176, 29.2688) -> (25.8658, 29.2528) centre (25.8417, 29.2608) ccw
  arc A874 (26.2553, 30.4212) -> (26.2071, 30.4372) centre (26.2312, 30.4292) ccw
  line L267 (25.8417, 29.2608) -> (26.2312, 30.4292)
  arc A875 (24.9428, 29.1564) -> (24.9428, 29.1056) centre (24.9428, 29.131) ccw
  arc A876 (25.4621, 29.1056) -> (25.4621, 29.1564) centre (25.4621, 29.131) ccw
  line L268 (24.9428, 29.131) -> (25.4621, 29.131)
  arc A877 (24.1357, 29.2354) -> (24.1357, 29.2862) centre (24.1357, 29.2608) ccw
  arc A878 (23.8111, 29.2862) -> (23.8111, 29.2354) centre (23.8111, 29.2608) ccw
  line L269 (24.1357, 29.2608) -> (23.8111, 29.2608)
  arc A879 (24.4856, 29.5854) -> (24.4348, 29.5854) centre (24.4602, 29.5854) ccw
  arc A880 (24.1357, 29.2862) -> (24.1357, 29.2354) centre (24.1357, 29.2608) ccw
  arc A881 (24.1357, 29.2608) -> (24.4602, 29.5854) centre (24.1356, 29.5854) ccw
  arc A882 (24.4856, 30.1046) -> (24.4348, 30.1046) centre (24.4602, 30.1046) ccw
  arc A883 (24.4348, 29.5854) -> (24.4856, 29.5854) centre (24.4602, 29.5854) ccw
  line L270 (24.4602, 30.1046) -> (24.4602, 29.5854)
  arc A884 (24.1357, 30.4546) -> (24.1357, 30.4038) centre (24.1357, 30.4292) ccw
  arc A885 (24.4348, 30.1046) -> (24.4856, 30.1046) centre (24.4602, 30.1046) ccw
  arc A886 (24.4602, 30.1046) -> (24.1357, 30.4292) centre (24.1356, 30.1046) ccw
  arc A887 (23.8111, 30.4546) -> (23.8111, 30.4038) centre (23.8111, 30.4292) ccw
  arc A888 (24.1357, 30.4038) -> (24.1357, 30.4546) centre (24.1357, 30.4292) ccw
  line L271 (23.8111, 30.4292) -> (24.1357, 30.4292)
  arc A889 (23.7857, 29.2608) -> (23.8365, 29.2608) centre (23.8111, 29.2608) ccw
  arc A890 (23.8365, 30.4292) -> (23.7857, 30.4292) centre (23.8111, 30.4292) ccw
  line L272 (23.8111, 29.2608) -> (23.8111, 30.4292)
  arc A891 (23.2156, 29.2608) -> (23.2664, 29.2608) centre (23.241, 29.2608) ccw
  arc A892 (23.2664, 30.4292) -> (23.2156, 30.4292) centre (23.241, 30.4292) ccw
  line L273 (23.241, 29.2608) -> (23.241, 30.4292)
  arc A893 (22.6141, 30.4415) -> (22.5697, 30.4169) centre (22.5919, 30.4292) ccw
  arc A894 (23.2188, 29.2485) -> (23.2632, 29.2731) centre (23.241, 29.2608) ccw
  line L274 (22.5919, 30.4292) -> (23.241, 29.2608)
  arc A895 (22.5665, 29.2608) -> (22.6173, 29.2608) centre (22.5919, 29.2608) ccw
  arc A896 (22.6173, 30.4292) -> (22.5665, 30.4292) centre (22.5919, 30.4292) ccw
  line L275 (22.5919, 29.2608) -> (22.5919, 30.4292)
  arc A897 (22.0275, 29.5275) -> (22.0275, 29.5783) centre (22.0275, 29.5529) ccw
  arc A898 (21.4433, 29.5783) -> (21.4433, 29.5275) centre (21.4433, 29.5529) ccw
  line L276 (22.0275, 29.5529) -> (21.4433, 29.5529)
  arc A899 (21.7595, 30.4372) -> (21.7113, 30.4212) centre (21.7354, 30.4292) ccw
  arc A900 (22.1007, 29.2528) -> (22.1489, 29.2688) centre (22.1248, 29.2608) ccw
  line L277 (21.7354, 30.4292) -> (22.1248, 29.2608)
  arc A901 (21.3218, 29.2688) -> (21.37, 29.2528) centre (21.3459, 29.2608) ccw
  arc A902 (21.7595, 30.4212) -> (21.7113, 30.4372) centre (21.7354, 30.4292) ccw
  line L278 (21.3459, 29.2608) -> (21.7354, 30.4292)
  line L279 (13.9293, 43.6118) -> (13.4777, 41.9862)
  arc A903 (20.447, 29.1564) -> (20.447, 29.1056) centre (20.447, 29.131) ccw
  arc A904 (20.9663, 29.1056) -> (20.9663, 29.1564) centre (20.9663, 29.131) ccw
  line L280 (20.447, 29.131) -> (20.9663, 29.131)
  arc A905 (19.8986, 29.7253) -> (19.923, 29.7699) centre (19.9108, 29.7476) ccw
  arc A906 (19.566, 29.9647) -> (19.5416, 29.9201) centre (19.5538, 29.9424) ccw
  line L281 (19.9108, 29.7476) -> (19.5538, 29.9424)
  arc A907 (19.9237, 29.7695) -> (19.8979, 29.7257) centre (19.9108, 29.7476) ccw
  arc A908 (20.0152, 29.5204) -> (20.066, 29.5204) centre (20.0406, 29.5204) ccw
  arc A909 (20.0406, 29.5204) -> (19.9108, 29.7476) centre (19.777, 29.5204) ccw
  arc A910 (19.5409, 29.9205) -> (19.5667, 29.9642) centre (19.5538, 29.9424) ccw
  arc A911 (19.4494, 30.1696) -> (19.3986, 30.1696) centre (19.424, 30.1696) ccw
  arc A912 (19.424, 30.1696) -> (19.5538, 29.9424) centre (19.6877, 30.1695) ccw